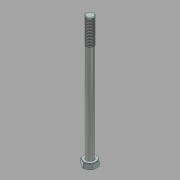
# Autodesk Inventor part: Hex Head Cap Screw
Saved by Autodesk Inventor 2011 SP2 (Build 150309200, 309)
## iProperties
Created: 2014-10-30
Part Number: Hex Head Cap Screw
Document SubType Name: Modeling
Designer: Greg Pavlik
Density: 1 g/cm^3
Author: Greg Pavlik
Autodesk Inventor part; units mm, degrees
ref_plane "YZ Plane" through (0, 0, 0) normal (1, 0, 0) x (0, 1, 0)
ref_plane "XZ Plane" through (0, 0, 0) normal (0, 1, 0) x (-1, 0, 0)
ref_plane "XY Plane" through (0, 0, 0) normal (0, 0, 1) x (1, 0, 0)
sketch "Sketch1" plane through (0, 0, 0) normal (0, 0, 1) x (1, 0, 0)
  circle A0 centre (0, 0) radius 1.5
  dimension "Diameter" = 3
  constraints: 1 centre point, 1 coincident
  measures "Diameter" diameter of A0
extrude "Extrusion1" add sketch "Sketch1" along normal blind 48
sketch "Sketch2" plane through (0, 0, 0) normal (0, 0, -1) x (-1, 0, 0)
  circle A0 centre (0, 0) radius 1.5 construction
  circle A1 centre (0, 0) radius 2.25
  dimension "Head_Washer_Diameter" = 4.5
  constraints: 1 centre point, 1 coincident
  measures "Head_Washer_Diameter" diameter of A1
extrude "Extrusion2" add sketch "Sketch2" along normal blind 0.25
sketch "Sketch3" plane through (0, 0, -0.25) normal (0, 0, -1) x (-1, 0, 0)
  circle A0 centre (0, 0) radius 2.25 construction
  line L0 (-2.25, 1.299) -> (0, 2.5981)
  line L1 (0, 2.5981) -> (2.25, 1.299)
  line L2 (2.25, 1.299) -> (2.25, -1.299)
  line L3 (2.25, -1.299) -> (0, -2.5981)
  line L4 (0, -2.5981) -> (-2.25, -1.299)
  line L5 (-2.25, -1.299) -> (-2.25, 1.299)
  constraints: 12 end point, 1 coincident, 1 tangent, 1 vertical, 13 other
extrude "Extrusion3" add sketch "Sketch3" along normal blind 2.001
thread "Thread1" size "M3x0.5" class "6g" standard "ANSI Metric M Profile" length 10
chamfer "Chamfer1" distance 0.25 angle 45 1 edges at (-1.5, 0, 48)
sketch "Sketch4" plane through (0, 0, 0) normal (0, 1, 0) x (-1, 0, 0)
  line L0 (-2.25, -0.25) -> (-2.25, -2.251) construction
  line L1 (-2.25, -0.25) -> (-2.25, -2.251) construction
  line L2 (-2.25, -2.251) -> (-3.45, -2.251)
  line L3 (-3.45, -2.251) -> (-3.45, -1.5582)
  line L4 (-3.45, -1.5582) -> (-2.25, -2.251)
  line L5 (0, 0) -> (0, -6.83)
  point P0 (-2.25, -0.25)
  dimension "Head_Chamfer_Angle" = 30
  dimension "d14" = 1.2
  constraints: 8 end point, 2 perpendicular, 1 parallel
  measures "Head_Chamfer_Angle" angle of L4 L2
  measures "d14" distance between parallel lines of L3 L0
revolve "Revolution1" cut sketch "Sketch4" angle 360 about axis through (0, 0, 0) along (0, 0, -1)
equation "\"Head_Washer_Diameter\" = 1.5 * Diameter"
equation "\"Head_Height\" = 0.667 * Diameter"
equation "\"d14\" = 0.4 * Diameter"
body "Solid1"
